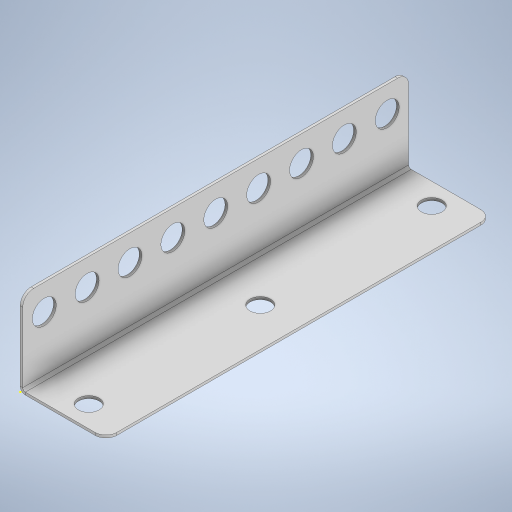
# Autodesk Inventor part: Mounting_bracket
Saved by Autodesk Inventor 2023 (Build 270158000, 158)
## iProperties
Created: 2023-04-20
Part Number: Mounting_bracket
Material: Generic
Document SubType Name: Sheet Metal
Designer: kaspe
Density: 1 g/cm^3
Sheet Metal Rule: Default_mm
Appearance: Default
Sheet Metal Width: 97,393 mm
Sheet Metal Length: 225,000 mm
Sheet Metal Area: 21913,407 mm^2
Flat Pattern Width: 9.73929 cm
Flat Pattern Length: 22.5 cm
Flat Pattern Area: 219.134 cm^2
Author: kaspe
Autodesk Inventor part; units mm, degrees
ref_plane "YZ Plane" through (0, 0, 0) normal (1, 0, 0) x (0, 1, 0)
ref_plane "XZ Plane" through (0, 0, 0) normal (0, 1, 0) x (-1, 0, 0)
ref_plane "XY Plane" through (0, 0, 0) normal (0, 0, 1) x (1, 0, 0)
sketch "Sketch2" plane through (0, 0, 0) normal (1, 0, 0) x (0, 1, 0)
  line L0 (0, 0) -> (50, 0)
  line L1 (50, 0) -> (50, -225)
  line L2 (50, -225) -> (0, -225)
  line L3 (0, -225) -> (0, 0)
  dimension "d0" = 50
  dimension "d1" = 225
  measures "d0" distance of L1.end L2.end
  measures "d1" distance of L0.end L1.end
extrude "Plate1" add sketch "Sketch2" along normal blind 1.5
sketch "Sketch3" plane through (0, 1.5, -225) normal (0, -1, 0) x (1, 0, 0)
  line L0 (0, 225) -> (0, 0)
  line L1 (0, 0) -> (25.4, 0)
  line L2 (25.4, 0) -> (25.4, 225)
  line L3 (25.4, 225) -> (0, 225)
  constraints: 6 end point, 1 horizontal, 1 perpendicular, 1 vertical
edge flange "Flange1" height 25.4 angle 90 thickness 1.5 bend radius 1.5 thickness toward (0, -1, 0) relief tear relief width 1.5 relief depth 0.75 edges at (1.5, 0, -112.5) wall of the first edge with corners at (0, 1.5, 0) (0, 1.5, -225) (25.4, 1.5, -225) (25.4, 1.5, 0)
bend "Bend1"
corner "Corner1"
sketch "Sketch4" plane through (25.4, 1.5, 0) normal (0, 1, 0) x (1, 0, 0)
  line L0 (-25.4, 0) -> (24.6, 0)
  line L1 (-22.4, 0) -> (0, 0)
  line L2 (-25.4, 0) -> (24.6, 0) construction
  line L3 (0, 225) -> (-22.4, 225)
  line L4 (24.6, 0) -> (-22.4, 0)
  line L5 (-22.4, 0) -> (-22.4, 225)
  line L6 (-22.4, 225) -> (24.6, 225)
  line L7 (24.6, 225) -> (24.6, 0)
  dimension "d13" = 50
  dimension "d14" = 0
  measures "d13" distance of L0.start L0.end
  measures "d14" distance between parallel lines of L2 L0
sheet face with bend "Face2" sketch "Sketch4" thickness 1.5 toward (0, -1, 0) bend radius 1.5
bend "Bend2"
sketch "Sketch5" plane through (0, 50, 0) normal (0, 0, 1) x (1, 0, 0)
  point P0 (0, -50)
sketch "Sketch6" plane through (3, 1.5, 0) normal (0, 1, 0) x (1, 0, 0)
  line L0 (47, 225) -> (47, 0) projected
  line L1 (0, 0) -> (47, 0) projected
  line L2 (47, 225) -> (24.5, 225)
  line L3 (24.5, 225) -> (24.5, 0)
  line L4 (24.5, 0) -> (47, 0)
  line L5 (47, 0) -> (47, 225)
  circle A0 centre (24.5, 112.5) radius 6
  line L6 (24.5, 112.5) -> (24.5, 12.5)
  line L7 (24.5, 112.5) -> (124.5, 112.5) construction
  line L8 (24.5, 112.5) -> (24.5, 212.5)
  line L9 (24.5, 112.5) -> (124.5, 112.5) construction
  circle A1 centre (24.5, 212.5) radius 6
  circle A2 centre (24.5, 12.5) radius 6
  point P0 (-3, 0)
  dimension "d20" = 22.5
  dimension "d21" = 12
  dimension "d22" = 100
  dimension "d23" = 90
  dimension "d24" = 100
  dimension "d25" = 90
  dimension "d26" = 12
  dimension "d27" = 12
  constraints: 16 end point, 3 centre point, 3 horizontal, 3 perpendicular, 2 coincident, 2 collinear, 2 parallel, 1 midpoint, 1 point on line
  measures "d20" distance of L4.end L3.end
  measures "d21" diameter of A0
  measures "d22" distance of L6.start L6.end
  measures "d23" angle of L6 L7
  measures "d24" distance of L6.start L8.end
  measures "d25" angle of L9 L8
  measures "d26" diameter of A1
  measures "d27" diameter of A2
hole "Hole1" at (27.5, 1.5, -12.5) at (27.5, 1.5, -112.5) at (27.5, 1.5, -212.5) direction (0, -1, 0) diameter 12 end through all clearance for "Flat Head Machine Screw" size "M10" standard "Ansi Metric M Profile"
fillet "Corner Round1" radius 6.35 4 edges at (50, 0.75, 0) (50, 0.75, -225) (0.75, 50, -225) (0.75, 50, 0)
sketch "Sketch7" plane through (1.5, 0, 0) normal (1, 0, 0) x (0, 0, -1)
  arc A0 (6.35, 50) -> (0, 43.65) centre (6.35, 43.65) ccw projected
  circle A1 centre (112.5, 35) radius 6.95
  line L0 (112.5, 35) -> (87.5, 35)
  line L1 (87.5, 35) -> (62.5, 35)
  line L2 (62.5, 35) -> (37.5, 35)
  line L3 (37.5, 35) -> (12.5, 35)
  circle A2 centre (12.5, 35) radius 6.95
  circle A3 centre (37.5, 35) radius 6.95
  circle A4 centre (62.5, 35) radius 6.95
  circle A5 centre (87.5, 35) radius 6.95
  line L4 (112.5, 35) -> (137.5, 35)
  line L5 (137.5, 35) -> (162.5, 35)
  line L6 (162.5, 35) -> (187.5, 35)
  line L7 (187.5, 35) -> (212.5, 35)
  circle A6 centre (137.5, 35) radius 6.95
  circle A7 centre (162.5, 35) radius 6.95
  circle A8 centre (187.5, 35) radius 6.95
  circle A9 centre (212.5, 35) radius 6.95
  point P0 (0, 0)
  dimension "d38" = 13.9
  dimension "d43" = 25
  dimension "d44" = 25
  dimension "d45" = 25
  dimension "d46" = 25
  dimension "d47" = 13.9
  dimension "d48" = 13.9
  dimension "d49" = 13.9
  dimension "d50" = 13.9
  dimension "d51" = 25
  dimension "d52" = 25
  dimension "d53" = 25
  dimension "d54" = 180
  dimension "d55" = 25
  dimension "d56" = 13.9
  dimension "d57" = 13.9
  dimension "d58" = 13.9
  dimension "d59" = 13.9
  constraints: 16 end point, 9 centre point, 8 coincident, 2 point on line, 1 collinear, 1 horizontal
  measures "d38" diameter of A1
  measures "d43" distance of L0.start L0.end
  measures "d44" distance of L0.end L1.end
  measures "d45" distance of L1.end L2.end
  measures "d46" distance of L2.end L3.end
  measures "d47" diameter of A2
  measures "d48" diameter of A3
  measures "d49" diameter of A4
  measures "d50" diameter of A5
  measures "d51" distance of L0.start L4.end
  measures "d52" distance of L4.end L5.end
  measures "d53" distance of L5.end L6.end
  measures "d54" angle of L6 L5
  measures "d55" distance of L6.end L7.end
  measures "d56" diameter of A6
  measures "d57" diameter of A7
  measures "d58" diameter of A8
  measures "d59" diameter of A9
hole "Hole2" at (1.5, 35, -12.5) at (1.5, 35, -37.5) at (1.5, 35, -62.5) at (1.5, 35, -87.5) at (1.5, 35, -112.5) at (1.5, 35, -137.5) at (1.5, 35, -162.5) at (1.5, 35, -187.5) at (1.5, 35, -212.5) direction (-1, 0, 0) diameter 13.9 end through all
equation "\"d2\" = Thickness"
equation "\"d3\" = BendReliefWidth"
equation "\"d4\" = BendReliefDepth"
equation "\"d5\" = MinimumRemnant"
equation "\"d6\" = TransitionRadius"
equation "\"d9\" = BendRadius"
equation "\"d10\" = CornerReliefSize"
equation "\"d11\" = GapSize"
equation "\"d12\" = JacobiRadiusSize"
equation "\"d15\" = BendRadius"
equation "\"d16\" = BendReliefWidth"
equation "\"d18\" = MinimumRemnant"
equation "\"d17\" = BendReliefDepth"
equation "\"d19\" = TransitionRadius"
equation "\"BendRadius\" = Thickness"
equation "\"BendReliefWidth\" = Thickness"
equation "\"BendReliefDepth\" = 0.5 * Thickness"
equation "\"CornerReliefSize\" = 4 * Thickness"
equation "\"MinimumRemnant\" = 2 * Thickness"
equation "\"TransitionRadius\" = BendRadius"
equation "\"JacobiRadiusSize\" = BendRadius"
equation "\"GapSize\" = Thickness"
equation "\"Thickness\" = 1.5"
body "Solid1"
